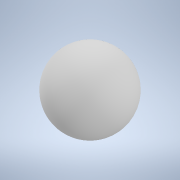
# Autodesk Inventor part: ball
Saved by Autodesk Inventor 2021 (Build 250183000, 183)
## iProperties
Created: 2021-07-07
Part Number: ball
Material: Generic
Document SubType Name: Modeling
Designer: Priyanka Hungund
Density: 1 g/cm^3
Appearance: Default
Author: Priyanka Hungund
Autodesk Inventor part; units mm, degrees
ref_plane "YZ Plane" through (0, 0, 0) normal (1, 0, 0) x (0, 1, 0)
ref_plane "XZ Plane" through (0, 0, 0) normal (0, 1, 0) x (-1, 0, 0)
ref_plane "XY Plane" through (0, 0, 0) normal (0, 0, 1) x (1, 0, 0)
sketch "Sketch1" plane through (0, 0, 0) normal (0, 0, 1) x (1, 0, 0)
  circle A0 centre (0, 0) radius 2.2511
  line L0 (-2.2511, 0) -> (2.2511, 0)
  dimension "d0" = 90
  constraints: 2 end point, 2 point on circle, 1 centre point, 1 coincident, 1 horizontal
revolve "Revolution1" add sketch "Sketch1" angle 360 about axis through (-2.2511, 0, 0) along (1, 0, 0) picked at (0.6644, 0.3487) contours L0 A0
body "Solid1"
